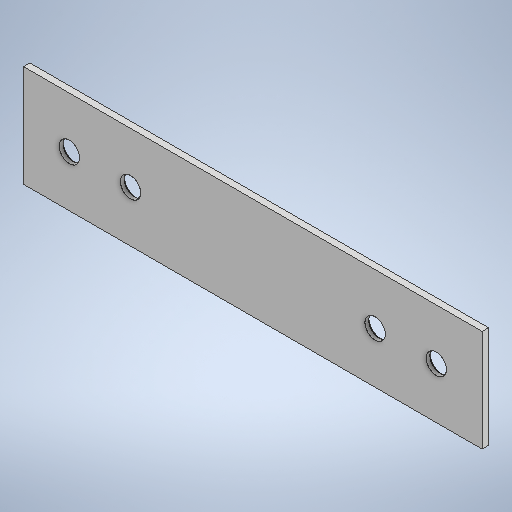
# Autodesk Inventor part: lacznik_plaski_180_40_2p5
Saved by Autodesk Inventor 2025.2 (Build 292293000, 293)
## iProperties
Created: 2025-03-18
Part Number: lacznik_plaski_180_40_2p5
Material: Ogólny
Document SubType Name: Modeling
Designer: tadek
Density: 1 g/cm^3
Appearance: Domyślna
Author: tadek
Autodesk Inventor part; units mm, degrees
ref_plane "YZ Plane" through (0, 0, 0) normal (1, 0, 0) x (0, 1, 0)
ref_plane "XZ Plane" through (0, 0, 0) normal (0, 1, 0) x (-1, 0, 0)
ref_plane "XY Plane" through (0, 0, 0) normal (0, 0, 1) x (1, 0, 0)
sketch "Szkic1" plane through (0, 0, 0) normal (0, 0, 1) x (1, 0, 0)
  line L0 (0, 0) -> (180, 0)
  line L1 (180, 0) -> (180, 40)
  line L2 (180, 40) -> (0, 40)
  line L3 (0, 40) -> (0, 0)
  line L4 (0, 20) -> (180, 20) construction
  line L5 (90, 0) -> (90, 40) construction
  line L6 (45, 0) -> (45, 40) construction
  line L7 (18, 40) -> (18, 0) construction
  circle A0 centre (18, 20) radius 4
  line L8 (30, 40) -> (30, 0) construction
  circle A1 centre (42, 20) radius 4
  circle A2 centre (162, 20) radius 4
  circle A3 centre (138, 20) radius 4
  dimension "d0" = 180
  dimension "d1" = 40
  dimension "d2" = 45
  dimension "d3" = 18
  dimension "d5" = 8
  dimension "d6" = 30
  constraints: 18 end point, 6 perpendicular, 6 point on line, 5 midpoint, 4 centre point, 3 symmetric about line, 1 horizontal, 3 other
  measures "d0" distance of L0.start L0.end
  measures "d1" distance of L0.end L1.end
  measures "d2" distance between parallel lines of L6 L3
  measures "d3" distance between parallel lines of L3 L7
  measures "d5" diameter of A0
  measures "d6" distance between parallel lines of L3 L8
extrude "Wyciągnięcie proste1" add sketch "Szkic1" along normal blind 2.5 contours L3 L2 L1 L0 | A0 | A1 | A2 | A3
hole "Otwór2" at (18, 20, 0) at (42, 20, 0) at (138, 20, 0) at (162, 20, 0) direction (0, 0, 1) diameter 8 end through all countersink diameter 10 countersink angle 90
